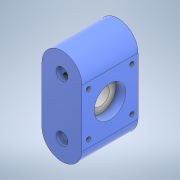
# Autodesk Inventor part: free_wheel_connector
Saved by Autodesk Inventor 2021 (Build 250183000, 183)
## iProperties
Created: 2020-10-27
Part Number: free_wheel_connector
Material: Generic
Document SubType Name: Modeling
Designer: Mateusz
Density: 1 g/cm^3
Appearance: Default
Author: Mateusz
Autodesk Inventor part; units mm, degrees
ref_plane "YZ Plane" through (0, 0, 0) normal (1, 0, 0) x (0, 1, 0)
ref_plane "XZ Plane" through (0, 0, 0) normal (0, 1, 0) x (-1, 0, 0)
ref_plane "XY Plane" through (0, 0, 0) normal (0, 0, 1) x (1, 0, 0)
sketch "Sketch1" plane through (0, 0, 0) normal (1, 0, 0) x (0, 1, 0)
  circle A0 centre (0, 0) radius 4.25
  line L0 (0, -20) -> (20, -20)
  line L1 (20, -20) -> (-20, -20)
  line L2 (20, -20) -> (35, -20)
  line L3 (-20, -20) -> (-35, -20)
  line L4 (-35, -20) -> (-35, 20)
  line L5 (-35, 20) -> (35, 20)
  line L6 (35, 20) -> (35, -20)
  circle A1 centre (0, 0) radius 11.25
  circle A2 centre (0, 0) radius 13
  dimension "d0" = 8.5
  dimension "d1" = 20
  dimension "d2" = 20
  dimension "d3" = 40
  dimension "d4" = 15
  dimension "d5" = 15
  dimension "d6" = 40
  dimension "d7" = 22.5
  dimension "d10" = 26
  constraints: 14 end point, 3 centre point, 3 coincident, 3 perpendicular, 2 point on line, 1 horizontal
  measures "d0" diameter of A0
  measures "d1" distance of A0.centre L0.start
  measures "d2" distance of L0.start L0.end
  measures "d3" distance of L0.end L1.end
  measures "d4" distance of L0.end L2.end
  measures "d5" distance of L1.end L3.end
  measures "d6" distance of L3.end L4.end
  measures "d7" diameter of A1
  measures "d10" diameter of A2
extrude "Extrusion1" add sketch "Sketch1" along normal blind 3 contours L1 L3 L4 L5 L6 L2 L0 | A2
sketch "Sketch2" plane through (0, -35, -20) normal (0, 0, -1) x (-1, 0, 0)
  line L0 (0, 70) -> (-3, 70) projected
  line L1 (0, 70) -> (0, 0) projected
  line L2 (0, 0) -> (11.25, 0)
  line L3 (22.5, 70) -> (22.5, 0)
  line L4 (22, 0) -> (0, 0)
  line L5 (25.5, 70) -> (25.5, 0)
  line L6 (25, 0) -> (22, 0)
  line L7 (0, 70) -> (22.5, 70)
  line L8 (22.5, 70) -> (25.5, 70)
  line L9 (22.5, 0) -> (25.5, 0)
  line L10 (0, 70) -> (11.25, 70)
  line L11 (11.25, 70) -> (11.25, 0)
  line L12 (0, 70) -> (0, 55)
  line L13 (0, 0) -> (0, 15)
  circle A0 centre (11.25, 15) radius 11.25
  circle A1 centre (11.25, 55) radius 11.25
  line L14 (-3, 70) -> (-3, 0) projected
  circle A2 centre (11.25, 55) radius 4.25
  circle A3 centre (11.25, 15) radius 4.25
  arc A4 (0, 6.2536) -> (22.5, 6.2536) centre (11.25, 15) ccw
  arc A5 (22.5, 23.7464) -> (0, 23.7464) centre (11.25, 15) ccw
  arc A6 (22.5, 63.7464) -> (0, 63.7464) centre (11.25, 55) ccw
  arc A7 (0, 46.2536) -> (22.5, 46.2536) centre (11.25, 55) ccw
  point P0 (0, 35)
  point P1 (22.5, 55)
  point P2 (22.5, 15)
  dimension "d27" = 11.25
  dimension "d28" = 15
  dimension "d29" = 15
  dimension "d30" = 8.5
  dimension "d31" = 8.5
  constraints: 24 end point, 10 point on line, 8 centre point, 8 point on circle, 4 coincident, 4 tangent, 3 perpendicular, 2 collinear, 2 horizontal, 1 midpoint, 1 vertical
  measures "d27" distance of L0.start L10.end
  measures "d28" distance of L0.start L12.end
  measures "d29" distance of L1.end L13.end
  measures "d30" diameter of A2
  measures "d31" diameter of A3
extrude "Extrusion3" add sketch "Sketch2" against normal up to surface (40 mm away) contours L8 L5 L9 L6 L3
extrude "Extrusion5" add sketch "Sketch2" against normal blind 3 contours L7 L11 A6 L1 | A6 L11 A1 L1 | L7 L3 A6 L11 | A1 L11 A7 L1 | A6 L3 A1 L11 | A7 L11 A5 L1 | A1 L3 A7 L11 | A5 L11 A0 L1 | A7 L3 A5 L11 | A0 L11 A4 L1 | A5 L3 A0 L11 | A4 L11 L2 L1 | A0 L3 A4 L11 | L6 L4 L11 A4 L3
sketch "Sketch3" plane through (-22.5, -35, 20) normal (1, 0, 0) x (0, 0, -1)
  circle A0 centre (20, 35) radius 11.25
  circle A1 centre (20, 35) radius 11.25 projected
  circle A2 centre (20, 35) radius 4.25
  dimension "d34" = 8.5
  constraints: 2 centre point, 2 coincident
  measures "d34" diameter of A2
extrude "Extrusion6" cut sketch "Sketch3" against normal up to surface (3 mm away) contours A0 | A2
sketch "Sketch4" plane through (-25.5, 35, 20) normal (0, 0, 1) x (1, 0, 0)
  circle A0 centre (14.25, -15) radius 4.25 projected
  arc A1 (25.5, -15) -> (3, -15) centre (14.25, -15) ccw projected
  arc A2 (3, -15) -> (25.5, -15) centre (14.25, -15) ccw projected
  arc A3 (25.5, -55) -> (3, -55) centre (14.25, -55) ccw projected
  arc A4 (3, -55) -> (25.5, -55) centre (14.25, -55) ccw projected
  line L0 (25.5, 0) -> (25.5, -70) projected
  line L1 (3, -70) -> (25.5, -70) projected
  line L2 (3, 0) -> (3, -70) projected
  line L3 (25.5, 0) -> (3, 0) projected
  point P0 (25.5, -35)
extrude "Extrusion7" add sketch "Sketch4" against normal blind 3 contours L0 A3 L2 A2 | A1 L2 L3 L0 | L0 L1 L2 A4
sketch "Sketch5" plane through (3, 35, 20) normal (0, 1, 0) x (1, 0, 0)
  line L0 (-25.5, 37) -> (-25.5, 3) projected
  line L1 (-25.5, 3) -> (-3, 3) projected
  line L2 (-25.5, 37) -> (-25.5, 3)
  line L3 (-25.5, 3) -> (-3, 3)
  line L4 (-3, 3) -> (-3, 37) projected
  line L5 (-3, 3) -> (-3, 37)
  line L6 (-3, 37) -> (-25.5, 37)
  point P0 (-3, 20)
  constraints: 8 end point, 3 perpendicular, 1 collinear
extrude "Extrusion8" add sketch "Sketch5" against normal up to surface (70 mm away)
extrude "Extrusion9" cut sketch "Sketch2" against normal up to surface (40 mm away) contours A2 L11 | L11 A2 | A3 L11 | L11 A3
extrude "Extrusion10" cut sketch "Sketch1" against normal up to surface (25.5 mm away) contours A0
sketch "Sketch6" plane through (3, -35, -20) normal (0, 0, -1) x (-1, 0, 0)
  circle A0 centre (14.25, 55) radius 4.25 projected
  circle A1 centre (14.25, 55) radius 14.25
  line L0 (28.5, 0) -> (28.5, 70) projected
  circle A2 centre (14.25, 15) radius 4.25 projected
  circle A3 centre (14.25, 15) radius 14.2824
  line L1 (28.5, 70) -> (0, 70) projected
  line L2 (0, 0) -> (0, 70) projected
  line L3 (28.5, 0) -> (0, 0) projected
  line L4 (28.5, 0) -> (28.5, 70) projected
  circle A4 centre (14.25, 55) radius 11.25 projected
  circle A5 centre (14.25, 15) radius 11.25 projected
  point P0 (3, 35)
  point P1 (28.5, 14.0382)
  point P2 (0, 14.0382)
  point P3 (0, 55)
  point P4 (28.5, 55)
  constraints: 2 centre point, 2 coincident, 1 tangent
extrude "Extrusion11" cut sketch "Sketch6" against normal up to surface (40 mm away) contours A1 L2 L1 L0 | L0 L3 L2 A3
sketch "Sketch7" plane through (-11.25, 20, 17) normal (0, 0, 1) x (1, 0, 0)
  circle A0 centre (0, 0) radius 4.25 projected
  circle A1 centre (0, 0) radius 11.25 projected
  circle A2 centre (0, -40) radius 4.25 projected
  circle A3 centre (0, -40) radius 11.25 projected
  point P0 (11.25, -20)
extrude "Extrusion12" cut sketch "Sketch7" against normal blind 4
sketch "Sketch8" plane through (-11.25, 20, -17) normal (0, 0, -1) x (-1, 0, 0)
  circle A0 centre (0, 0) radius 4.25 projected
  circle A1 centre (0, 0) radius 11.25 projected
  circle A2 centre (0, -40) radius 4.25 projected
  circle A3 centre (0, -40) radius 11.25 projected
  point P0 (-11.25, -20)
extrude "Extrusion13" cut sketch "Sketch8" against normal blind 4
sketch "Sketch9" plane through (-11.25, 20, 13) normal (0, 0, 1) x (1, 0, 0)
  circle A0 centre (0, 0) radius 11.25 projected
  circle A1 centre (0, 0) radius 4.25 projected
  circle A2 centre (0, -40) radius 11.25 projected
  circle A3 centre (0, -40) radius 4.25 projected
  point P0 (11.25, -20)
extrude "Extrusion14" add sketch "Sketch9" along normal up to surface (7 mm away)
sketch "Sketch10" plane through (-11.25, 20, -13) normal (0, 0, -1) x (-1, 0, 0)
  circle A0 centre (0, 0) radius 11.25 projected
  circle A1 centre (0, 0) radius 4.25 projected
  circle A2 centre (0, -40) radius 11.25 projected
  circle A3 centre (0, -40) radius 4.25 projected
  point P0 (-11.25, -20)
extrude "Extrusion15" add sketch "Sketch10" along normal up to surface (7 mm away)
sketch "Sketch11" plane through (0, 0, 0) normal (1, 0, 0) x (0, 0, -1)
  circle A0 centre (0, 0) radius 4.25 projected
  circle A1 centre (0, 0) radius 11.25 projected
extrude "Extrusion16" cut sketch "Sketch11" against normal blind 4
sketch "Sketch12" plane through (-22.5, 0, 0) normal (-1, 0, 0) x (0, 0, 1)
  circle A0 centre (0, 0) radius 4.25 projected
  circle A1 centre (0, 0) radius 11.25 projected
extrude "Extrusion17" cut sketch "Sketch12" against normal blind 4
sketch "Sketch13" plane through (3, 0, 0) normal (1, 0, 0) x (0, 0, -1)
  line L0 (0, 15.5) -> (-15.5, 15.5)
  line L1 (-15.5, 15.5) -> (-15.5, -15.5)
  line L2 (-15.5, -15.5) -> (15.5, -15.5)
  line L3 (15.5, -15.5) -> (15.5, 15.5)
  line L4 (15.5, 15.5) -> (0, 15.5)
  circle A0 centre (-15.5, 15.5) radius 1.45
  circle A1 centre (-15.5, -15.5) radius 1.45
  circle A2 centre (15.5, -15.5) radius 1.45
  circle A3 centre (15.5, 15.5) radius 1.45
  point P0 (0, 0)
  dimension "d59" = 15.5
  dimension "d60" = 15.5
  dimension "d61" = 31
  dimension "d62" = 31
  dimension "d63" = 31
  dimension "d64" = 2.9
  dimension "d65" = 2.9
  dimension "d66" = 2.9
  dimension "d67" = 2.9
  constraints: 10 end point, 4 centre point, 4 coincident, 2 perpendicular, 1 horizontal, 1 point on line
  measures "d59" distance of point (0, 0) L0.start
  measures "d60" distance of L0.start L0.end
  measures "d61" distance of L0.end L1.end
  measures "d62" distance of L1.end L2.end
  measures "d63" distance of L2.end L3.end
  measures "d64" diameter of A0
  measures "d65" diameter of A1
  measures "d66" diameter of A2
  measures "d67" diameter of A3
extrude "Extrusion18" cut sketch "Sketch13" against normal through all contours A0 L1 L0 | L0 L1 A0 | A3 L3 L4 | L4 L3 A3 | A1 L2 L1 | L1 L2 A1 | A2 L2 L3 | L3 L2 A2
sketch "Sketch14" plane through (-18.5, 0, 0) normal (-1, 0, 0) x (0, 0, 1)
  circle A0 centre (0, 0) radius 4.25 projected
  circle A1 centre (0, 0) radius 6.5
  dimension "d70" = 13
  constraints: 1 centre point, 1 coincident
  measures "d70" diameter of A1
extrude "Extrusion19" cut sketch "Sketch14" against normal up to surface (14.5 mm away)
body "Solid1"
